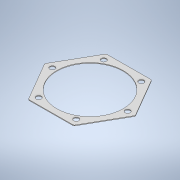
# Autodesk Inventor part: crankcase gasket
Saved by Autodesk Inventor 2020 (Build 240168000, 168)
## iProperties
Created: 2020-08-04
Part Number: crankcase gasket
Material: Generic
Document SubType Name: Modeling
Designer: benny
Density: 1 g/cm^3
Appearance: Default
Author: benny
Autodesk Inventor part; units mm, degrees
ref_plane "YZ Plane" through (0, 0, 0) normal (1, 0, 0) x (0, 1, 0)
ref_plane "XZ Plane" through (0, 0, 0) normal (0, 1, 0) x (-1, 0, 0)
ref_plane "XY Plane" through (0, 0, 0) normal (0, 0, 1) x (1, 0, 0)
sketch "Sketch3" plane through (0, 0, 0) normal (0, 1, 0) x (-1, 0, 0)
  circle A0 centre (0, 0) radius 53
  line L0 (-61.1985, -0.2718) -> (-30.8346, 52.8636)
  line L1 (-30.8346, 52.8636) -> (30.3639, 53.1354)
  line L2 (30.3639, 53.1354) -> (61.1985, 0.2718)
  line L3 (61.1985, 0.2718) -> (30.8346, -52.8636)
  line L4 (30.8346, -52.8636) -> (-30.3639, -53.1354)
  line L5 (-30.3639, -53.1354) -> (-61.1985, -0.2718)
  point P0 (-45.7812, -26.7036)
  dimension "d4" = 106
  constraints: 12 end point, 2 coincident, 1 midpoint, 16 other
extrude "Extrusion2" add sketch "Sketch3" along normal blind 1
sketch "Sketch4" plane through (0, 1, 0) normal (0, 1, 0) x (1, 0, 0)
  circle A0 centre (0, 0) radius 45
  dimension "d7" = 90
  constraints: 1 centre point, 1 coincident
  measures "d7" diameter of A0
extrude "Extrusion3" cut sketch "Sketch4" against normal blind 1
sketch "Sketch11" plane through (0, 1, 0) normal (0, 1, 0) x (1, 0, 0)
  line L0 (0, 0) -> (51, 0)
  circle A0 centre (51, 0) radius 3.5
  dimension "d19" = 51
  dimension "d20" = 7
  constraints: 2 end point, 1 centre point, 1 coincident, 1 horizontal
  measures "d19" distance of L0.start L0.end
  measures "d20" diameter of A0
extrude "Extrusion5" cut sketch "Sketch11" against normal blind 10
pattern_circular "Circular Pattern2" count 6 over 360 about axis through (0, 1, 0) along (0, -1, 0) of "Extrusion5"
fillet "Fillet1" radius 2 1 edges at (-30.3639, 0.5, 53.1354)
pattern_circular "Circular Pattern3" count 6 over 360 about axis through (0, 1, 0) along (0, -1, 0) of "Fillet1"
body "Solid2"
